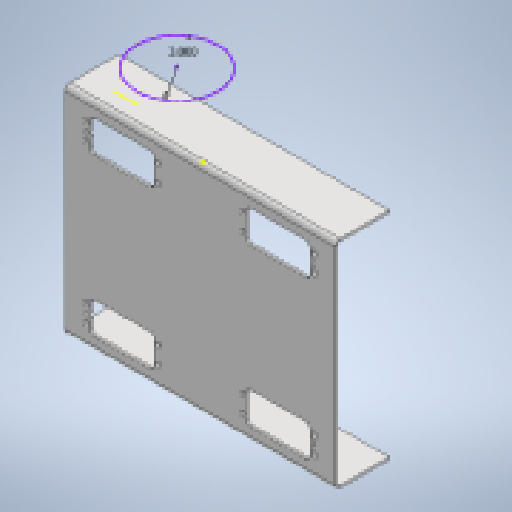
# Autodesk Inventor part: MainPlate
Saved by Autodesk Inventor 2024 (Build 280153000, 153)
## iProperties
Created: 2024-01-18
Part Number: MainPlate
Material: Generic
Document SubType Name: Sheet Metal
Designer: student
Density: 1 g/cm^3
Sheet Metal Rule: Default
Appearance: Default
Author: student
Autodesk Inventor part; units mm, degrees
note: some values were not read from the file. Chosen so that the rebuilt part matches the saved one: flange form of "Plate2".
ref_plane "YZ Plane" through (0, 0, 0) normal (1, 0, 0) x (0, 1, 0)
ref_plane "XZ Plane" through (0, 0, 0) normal (0, 1, 0) x (-1, 0, 0)
ref_plane "XY Plane" through (0, 0, 0) normal (0, 0, 1) x (1, 0, 0)
sketch "Sketch1" plane through (0, 0, 0) normal (0, 0, 1) x (1, 0, 0)
  line L0 (-152.4, 101.6) -> (152.4, 101.6)
  line L1 (152.4, 101.6) -> (152.4, -101.6)
  line L2 (152.4, -101.6) -> (-152.4, -101.6)
  line L3 (-152.4, -101.6) -> (-152.4, 101.6)
  line L4 (-152.4, 101.6) -> (152.4, -101.6) construction
  line L5 (152.4, 101.6) -> (-152.4, -101.6) construction
  point P0 (0, 0)
  dimension "d0" = 304.8
  dimension "d1" = 203.2
  measures "d0" distance of L1.end L2.end
  measures "d1" distance of L0.end L1.end
extrude "Plate1" add sketch "Sketch1" along normal blind 2.286
sketch "Sketch2" plane through (152.4, 99.314, 2.286) normal (0, 1, 0) x (-1, 0, 0)
  line L0 (304.8, 0) -> (0, 0)
  line L1 (0, 0) -> (0, -76.2)
  line L2 (0, -76.2) -> (304.8, -76.2)
  line L3 (304.8, -76.2) -> (304.8, 0)
  constraints: 6 end point, 1 horizontal, 1 perpendicular, 1 vertical
edge flange "Flange1" height 76.2 angle 90 thickness 2.286 bend radius 2.286 thickness toward (0, 1, 0) relief tear relief width 2.286 relief depth 1.143 corner gap 2.286 corner form 0 edges at (0, 101.6, 0) (0, -101.6, 0) wall of the first edge with corners at (-152.4, 99.314, 2.286) (152.4, 99.314, 2.286) (152.4, 99.314, -73.914) (-152.4, 99.314, -73.914)
bend "Bend1"
corner "Corner1"
sketch "Sketch3" plane through (-152.4, 101.6, -73.914) normal (0, 1, 0) x (1, 0, 0)
  point P0 (152.4, -73.914)
sketch "Sketch5" plane through (0, 0, 0) normal (0, 0, -1) x (-1, 0, 0)
  arc A0 (134.5614, 85.6) -> (134.5614, 82.8) centre (132.8, 84.2) ccw
  arc A1 (134.5614, 69.6) -> (134.5614, 66.8) centre (132.8, 68.2) ccw
  line L0 (128.3077, 75.4052) -> (132.4, 75.4052)
  arc A2 (132.4, 75.4052) -> (132.4, 77.0052) centre (132.4, 76.2052) ccw
  line L1 (132.4, 77.0052) -> (128.3077, 77.0052)
  arc A3 (69.2925, 64.909) -> (72.4991, 61.7024) centre (72.4991, 64.909) ccw
  line L2 (69.2922, 87.5) -> (69.2925, 64.909)
  arc A4 (72.4999, 90.7077) -> (69.2922, 87.5) centre (72.4999, 87.5) ccw
  line L3 (125.1, 90.7077) -> (72.4999, 90.7077)
  arc A5 (128.3077, 87.5) -> (125.1, 90.7077) centre (125.1, 87.5) ccw
  arc A6 (124.9841, 61.6858) -> (128.3077, 64.7165) centre (125.2346, 64.7488) ccw
  line L4 (124.9841, 61.6858) -> (72.5003, 61.7024)
  line L5 (128.3077, 64.7165) -> (128.3077, 75.4052)
  line L6 (128.3077, 77.0052) -> (128.3077, 87.5)
  circle A7 centre (132.8, 68.2) radius 2.25
  circle A8 centre (132.8, 84.2) radius 2.25
  circle A9 centre (64.8, 84.2) radius 2.25
  circle A10 centre (64.8, 68.2) radius 2.25
  arc A11 (68.6575, 64.9089) -> (72.4956, 61.0674) centre (72.4991, 64.909) ccw
  line L7 (68.6575, 64.9089) -> (68.6572, 87.5)
  arc A12 (72.4999, 91.3427) -> (68.6572, 87.5) centre (72.4999, 87.5) ccw
  line L8 (72.4999, 91.3427) -> (125.1, 91.3427)
  arc A13 (128.9427, 87.5) -> (125.1, 91.3427) centre (125.1, 87.5) ccw
  line L9 (128.9427, 87.5) -> (128.9427, 77.6402)
  line L10 (128.9427, 77.6402) -> (132.4, 77.6402)
  circle A14 centre (64.8, 84.2) radius 2.631
  circle A15 centre (64.8, 68.2) radius 2.631
  circle A16 centre (132.8, 68.2) radius 2.631
  circle A17 centre (132.8, 84.2) radius 2.631
  arc A18 (132.4, 74.7702) -> (132.4, 77.6402) centre (132.4, 76.2052) ccw
  line L11 (132.4, 74.7702) -> (128.9427, 74.7702)
  line L12 (128.9427, 74.7702) -> (128.9427, 64.7134)
  arc A19 (124.9593, 61.0508) -> (128.9427, 64.7134) centre (125.2346, 64.7488) ccw
  line L13 (124.9593, 61.0508) -> (72.4956, 61.0674)
  arc A20 (63.0386, 66.8) -> (63.0386, 69.6) centre (64.8, 68.2) ccw
  arc A21 (63.0386, 82.8) -> (63.0386, 85.6) centre (64.8, 84.2) ccw
  circle A22 centre (114.3, 76.2) radius 2.159
  line L14 (152.4, 97.028) -> (152.4, -97.028) projected
  line L15 (152.4, 101.6) -> (-152.4, 101.6) projected
  point P0 (0, 0)
  dimension "d20" = 0.635
  dimension "d21" = 0.381
  dimension "d22" = 0.635
  dimension "d23" = 0.8
  dimension "d24" = 0
  dimension "d28" = 38.1
  dimension "d29" = 25.4
  constraints: 29 point on circle, 28 end point, 19 centre point, 2 coincident, 12 other
  measures "d20" radial gap between concentric circles of A4 A12
  measures "d22" distance between parallel lines of L13 L4
  measures "d23" radius of A2
  measures "d24" angle of L1 L0
  measures "d28" distance from line of L14 point (114.3, 76.2)
  measures "d29" distance from line of L15 point (114.3, 76.2)
extrude "Cut2" cut sketch "Sketch5" against normal blind 2.286 contours A8 A0 | A7 A1 | L5 A6 L4 A3 L2 A4 L3 A5 L6 L1 A2 L0 | A9 | A10 | L7 A12 L8 A13 L9 L10 A18 L11 L12 A19 L13 A11 | A14 | A15 | A16 | A17 | A22
mirror "Mirror1" about plane through (0, 0, 0) normal (0, 1, 0) of "Cut2"
mirror "Mirror3" about plane through (0, 0, 0) normal (1, 0, 0) of "Cut2", "Mirror1"
sketch "Sketch7" plane through (-152.4, 101.6, -73.914) normal (0, 1, 0) x (1, 0, 0)
  arc A0 (51.1475, -24.2944) -> (24.2196, -23.4615) centre (38.1, -10.414) ccw
  line L0 (0, -71.628) -> (0, 0) projected
  line L1 (0, -46.228) -> (24.2196, -23.4615)
  line L2 (51.1475, -24.2944) -> (71.7652, -46.228)
  line L3 (0, -71.628) -> (304.8, -71.628) projected
  line L4 (0, -73.914) -> (304.8, -73.914) projected
  line L5 (152.4, -73.914) -> (152.4, 39.1866)
  line L6 (71.7652, -46.228) -> (152.4, -46.228)
  arc A1 (280.5804, -23.4615) -> (253.6525, -24.2944) centre (266.7, -10.414) ccw
  line L7 (304.8, -46.228) -> (280.5804, -23.4615)
  line L8 (253.6525, -24.2944) -> (233.0348, -46.228)
  line L9 (233.0348, -46.228) -> (152.4, -46.228)
  line L10 (0, -71.628) -> (304.8, -71.628) projected
  line L11 (304.8, 0) -> (304.8, -71.628) projected
  line L12 (0, 0) -> (304.8, 0) projected
  line L13 (0, -71.628) -> (0, 0) projected
  point P0 (282.6515, 0)
  point P1 (250.7485, 0)
  point P2 (54.0515, 0)
  point P3 (22.1485, 0)
  dimension "d31" = 90
  dimension "d32" = 25.4
  dimension "d34" = 63.5
  constraints: 14 end point, 6 symmetric about line, 4 point on circle, 3 coincident, 2 centre point, 2 point on line, 1 horizontal alignment, 1 parallel, 1 vertical, 1 other
  measures "d31" angle of L1 L2
  measures "d32" distance from line of L1.start L3
  measures "d34" distance from line of A0.centre L4
extrude "Extrusion1" cut sketch "Sketch7" against normal through all contours A0 L12 L5 L6 L2 | A0 L1 L0 L12 | L12 A1 L8 L9 L5 | L12 L11 L7 A1
fillet "Corner Round1" radius 6.35 4 edges at (-152.4, 100.457, -27.686) (152.4, 100.457, -27.686) (-152.4, -100.457, -27.686) (152.4, -100.457, -27.686)
fillet "Corner Round2" radius 6.35 8 edges at (128.1804, 100.457, -50.4525) (101.2525, 100.457, -49.6196) (-101.2525, 100.457, -49.6196) (-128.1804, 100.457, -50.4525) (-128.1804, -100.457, -50.4525) (-101.2525, -100.457, -49.6196) (101.2525, -100.457, -49.6196) (128.1804, -100.457, -50.4525)
equation "\"d25\" = Thickness"
equation "\"d2\" = Thickness"
equation "\"d3\" = BendReliefWidth"
equation "\"d4\" = BendReliefDepth"
equation "\"d5\" = MinimumRemnant"
equation "\"d6\" = TransitionRadius"
equation "\"d9\" = BendRadius"
equation "\"d10\" = CornerReliefSize"
equation "\"d11\" = GapSize"
equation "\"d12\" = JacobiRadiusSize"
equation "\"BendRadius\" = Thickness"
equation "\"BendReliefWidth\" = Thickness"
equation "\"BendReliefDepth\" = 0.5 * Thickness"
equation "\"CornerReliefSize\" = 4 * Thickness"
equation "\"MinimumRemnant\" = 2 * Thickness"
equation "\"TransitionRadius\" = BendRadius"
equation "\"JacobiRadiusSize\" = BendRadius"
equation "\"GapSize\" = Thickness"
equation "\"Thickness\" = 2.286"
body "Solid1"
